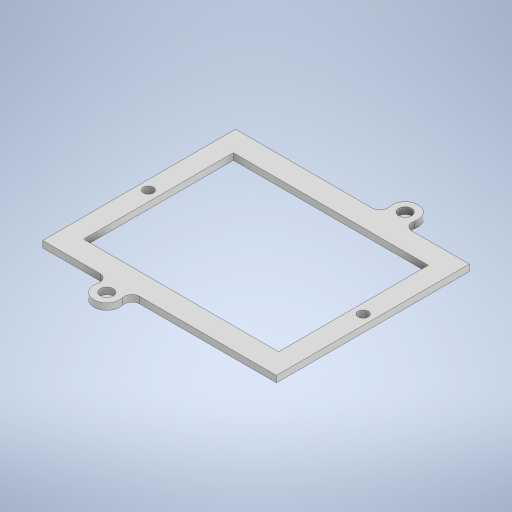
# Autodesk Inventor part: CO-1-06-fuseMountTop
Saved by Autodesk Inventor 2024 (Build 280153000, 153)
## iProperties
Created: 2023-03-23
Part Number: CO-1-06-fuseMountTop
Material: Generic
Document SubType Name: Modeling
Designer: beh5452
Density: 1 g/cm^3
Appearance: Default
Author: beh5452
Autodesk Inventor part; units mm, degrees
ref_plane "YZ Plane" through (0, 0, 0) normal (1, 0, 0) x (0, 1, 0)
ref_plane "XY Plane" through (0, 0, 0) normal (0, 0, 1) x (1, 0, 0)
ref_plane "Work Plane4" through (0, 32, 0) normal (0, 1, 0) x (-1, 0, 0)
sketch "Sketch1" plane through (0, 0, 0) normal (0, 1, 0) x (-1, 0, 0)
  line L0 (33.75, 44.75) -> (-33.75, 44.75)
  line L1 (-33.75, 44.75) -> (-33.75, -44.75)
  line L2 (-33.75, -44.75) -> (33.75, -44.75)
  line L3 (33.75, -44.75) -> (33.75, 44.75)
  line L4 (21.75, -36.75) -> (-21.75, -36.75)
  line L5 (21.75, 36.75) -> (-21.75, 36.75)
  line L6 (21.75, 36.75) -> (21.75, -36.75)
  line L7 (-21.75, 36.75) -> (-21.75, -36.75)
  line L8 (33.75, -41.75) -> (-33.75, -41.75)
  line L9 (33.75, 41.75) -> (-33.75, 41.75)
  line L10 (-6.7955, 36.75) -> (21.75, 0)
  line L11 (21.75, 0) -> (0, -36.75)
  point P0 (0, 0)
  point P1 (-33.75, 0)
  dimension "d0" = 83.5
  dimension "d1" = 3
  dimension "d2" = 3
  dimension "d4" = 5
  dimension "d5" = 5
  dimension "d6" = 12
  dimension "d7" = 12
  dimension "d8" = 67.5
  dimension "d9" = 33.75
  dimension "d10" = 41.75
  constraints: 24 end point, 7 perpendicular, 5 point on line, 3 horizontal, 3 midpoint
  measures "d0" distance between parallel lines of L8 L9
  measures "d1" distance between parallel lines of L0 L9
  measures "d2" distance between parallel lines of L8 L2
  measures "d4" distance between parallel lines of L9 L5
  measures "d5" distance between parallel lines of L8 L4
  measures "d6" distance between parallel lines of L3 L6
  measures "d7" distance between parallel lines of L7 L1
  measures "d8" distance from line of point (-33.75, 0) L3
  measures "d9" distance from line of point (0, 0) L1
  measures "d10" distance from line of point (0, 0) L8
sketch "Sketch2" plane through (0, 32, 0) normal (0, 1, 0) x (1, 0, 0)
  line L0 (-65.75, 34.75) -> (24.75, 34.75)
  line L1 (-65.75, -34.75) -> (24.75, -34.75)
  line L2 (24.75, -34.75) -> (24.75, 34.75)
  line L3 (-65.75, -34.75) -> (-65.75, 34.75)
  line L4 (-74.75, -44.75) -> (-74.75, 44.75)
  line L5 (33.75, -44.75) -> (33.75, 44.75) projected
  line L6 (33.75, 44.75) -> (-33.75, 44.75) projected
  line L7 (-74.75, -44.75) -> (33.75, -44.75)
  line L8 (-74.75, 44.75) -> (33.75, 44.75)
  dimension "d94" = 69.5
  dimension "d96" = 90.5
  dimension "d97" = 9
  dimension "d98" = 9
  dimension "d99" = 10
  dimension "d100" = 10
  constraints: 16 end point, 3 perpendicular, 2 point on line, 1 collinear
  measures "d94" distance between parallel lines of L0 L1
  measures "d96" distance between parallel lines of L2 L3
  measures "d97" distance between parallel lines of L2 L5
  measures "d98" distance between parallel lines of L4 L3
  measures "d99" distance between parallel lines of L7 L1
  measures "d100" distance between parallel lines of L8 L0
extrude "Extrusion3" add sketch "Sketch2" along normal blind 3
sketch "Sketch3" plane through (0, 32, 0) normal (0, 1, 0) x (1, 0, 0)
  circle A0 centre (29.25, 0) radius 4.5
  circle A1 centre (-70.45, 0) radius 4.5
  circle A2 centre (-70.45, 0) radius 2.35
  circle A3 centre (29.25, 0) radius 2.35
  line L0 (33.75, -44.75) -> (33.75, 44.75)
  point P0 (0, 0)
  dimension "d24" = 9
  dimension "d27" = 4.7
  dimension "d43" = 99.7
  dimension "d44" = 4.5
  constraints: 4 centre point, 2 coincident, 2 end point, 2 equal radius, 2 horizontal alignment
  measures "d24" diameter of A1
  measures "d27" diameter of A2
  measures "d43" distance of A1.centre A0.centre
  measures "d44" distance from line of L0 A0.centre
extrude "Extrusion5" cut sketch "Sketch3" along normal blind 3 contours A2 | A3
sketch "Sketch9" plane through (0, 35, 0) normal (0, 1, 0) x (1, 0, 0)
  circle A0 centre (-39, -50.75) radius 3
  circle A1 centre (-39, -50.75) radius 6
  line L0 (-74.75, -44.75) -> (33.75, -44.75) projected
  circle A2 centre (-2, -50.75) radius 3
  circle A3 centre (-2, -50.75) radius 6
  arc A4 (7.1652, -44.75) -> (3.7885, -49.1711) centre (7.1652, -48.25) ccw
  arc A5 (-7.7885, -49.1711) -> (-11.1652, -44.75) centre (-11.1652, -48.25) ccw
  arc A6 (-29.8348, -44.75) -> (-33.2115, -49.1711) centre (-29.8348, -48.25) ccw
  arc A7 (-44.7885, -49.1711) -> (-48.1652, -44.75) centre (-48.1652, -48.25) ccw
  line L1 (33.75, -44.75) -> (33.75, 44.75) projected
  line L2 (-74.75, 44.75) -> (-74.75, -44.75) projected
  line L3 (64.0405, 0) -> (-151.031, 0) construction
  circle A8 centre (-39, 50.75) radius 3
  circle A9 centre (-39, 50.75) radius 6
  circle A10 centre (-2, 50.75) radius 3
  circle A11 centre (-2, 50.75) radius 6
  arc A12 (3.7885, 49.1711) -> (7.1652, 44.75) centre (7.1652, 48.25) ccw
  arc A13 (-11.1652, 44.75) -> (-7.7885, 49.1711) centre (-11.1652, 48.25) ccw
  arc A14 (-33.2115, 49.1711) -> (-29.8348, 44.75) centre (-29.8348, 48.25) ccw
  arc A15 (-48.1652, 44.75) -> (-44.7885, 49.1711) centre (-48.1652, 48.25) ccw
  line L4 (33.75, 44.75) -> (-74.75, 44.75) projected
  point P0 (0, 0)
  dimension "d101" = 6
  dimension "d102" = 12
  dimension "d103" = 37
  dimension "d104" = 7
  dimension "d105" = 108.5
  dimension "d106" = 35.75
  constraints: 24 point on circle, 16 centre point, 16 symmetric about line, 10 tangent, 5 equal radius, 4 coincident, 4 point on line, 2 end point, 1 horizontal, 8 other
  measures "d101" diameter of A0
  measures "d102" diameter of A1
  measures "d103" distance of A0.centre A2.centre
  measures "d104" diameter of A7
  measures "d105" distance between parallel lines of L1 L2
  measures "d106" distance from line of L2 A0.centre
extrude "Extrusion10" add sketch "Sketch9" against normal blind 3 contours A1 | A1 L0 A6 | A7 L0 A1 | L4 A11 A12 | A13 A11 L4 | A11
equation "\"d9\" = 0.5 * d8"
equation "\"d10\" = 0.5 * d0"
equation "\"d44\" = 0.5 * d24"
equation "\"d2\" = d1"
equation "\"d5\" = d4"
equation "\"d7\" = d6"
body "Solid1"
